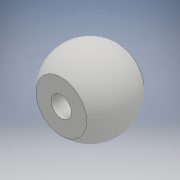
# Autodesk Inventor part: shifter ball
Saved by Autodesk Inventor 2017 (Build 210142000, 142)
## iProperties
Created: 2018-04-17
Part Number: shifter ball
Material: Generic
Document SubType Name: Modeling
Designer: RKL
Density: 1 g/cm^3
Appearance: Default
Author: RKL
Autodesk Inventor part; units mm, degrees
ref_plane "YZ Plane" through (0, 0, 0) normal (1, 0, 0) x (0, 1, 0)
ref_plane "XY Plane" through (0, 0, 0) normal (0, 0, 1) x (1, 0, 0)
sketch "Sketch1" plane through (0, 0, 0) normal (0, 0, 1) x (1, 0, 0)
  arc A0 (0, -12) -> (0, 12) centre (0, 0) ccw
  line L0 (0, 12) -> (0, -12)
  dimension "d0" = 24
  constraints: 2 coincident, 2 end point, 2 point on circle, 1 centre point, 1 midpoint, 1 vertical
  measures "d0" distance of L0.start L0.end
revolve "Revolution1" add sketch "Sketch1" angle 360 about axis through (0, 12, 0) along (0, -1, 0)
sketch "Sketch2" plane through (0, 0, 0) normal (0, 1, 0) x (-1, 0, 0)
  circle A0 centre (0, 0) radius 3.175
  dimension "d2" = 6.35
  constraints: 1 centre point, 1 coincident
  measures "d2" diameter of A0
extrude "Extrusion1" cut sketch "Sketch2" along normal through all both and the other way through all
ref_plane "Work Plane1" through (0, 12, 0) normal (0, 1, 0) x (-1, 0, 0)
sketch "Sketch3" plane through (0, 12, 0) normal (0, 1, 0) x (-1, 0, 0)
  circle A0 centre (0, 0) radius 12 projected
extrude "Extrusion2" cut sketch "Sketch3" against normal blind 3
mirror "Mirror1" about plane through (0, 0, 0) normal (0, 1, 0) of "Extrusion2"
body "Solid1"
